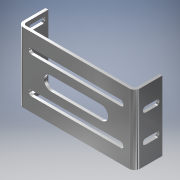
# Autodesk Inventor part: palmrest_cup
Saved by Autodesk Inventor 2018 (Build 220112000, 112)
## iProperties
Created: 2018-04-07
Part Number: palmrest_cup
Material: アルミニウム 6061
Document SubType Name: Sheet Metal
Designer: NaMACHAN
Density: 2.7 g/cm^3
Sheet Metal Rule: Default_mm
Appearance: アルミニウム - フラット
Mass: 33.0555 g
Surface Area: 100.911 cm^2
Volume: 12.2428 cm^3
Flat Pattern Width: 5 cm
Flat Pattern Length: 11.7048 cm
Flat Pattern Area: 58.5239 cm^2
Sheet Metal Width: 50.000 mm
Sheet Metal Length: 117.048 mm
Sheet Metal Area: 5852.389 mm^2
Author: NaMACHAN
Autodesk Inventor part; units mm, degrees
ref_plane "YZ Plane" through (0, 0, 0) normal (1, 0, 0) x (0, 1, 0)
ref_plane "XZ Plane" through (0, 0, 0) normal (0, 1, 0) x (-1, 0, 0)
ref_plane "XY Plane" through (0, 0, 0) normal (0, 0, 1) x (1, 0, 0)
sketch "スケッチ1" plane through (0, 0, 0) normal (0, 1, 0) x (-1, 0, 0)
  line L0 (-42, -25) -> (42, -25)
  line L1 (42, -25) -> (42, 25)
  line L2 (42, 25) -> (-42, 25)
  line L3 (-42, 25) -> (-42, -25)
  line L4 (-42, -25) -> (42, 25) construction
  line L5 (42, -25) -> (-42, 25) construction
  point P0 (0, 0)
  dimension "d0" = 84
  dimension "d1" = 50
  measures "d0" distance of L2.end L1.end
  measures "d1" distance of L1.end L0.end
extrude "プレート1" add sketch "スケッチ1" along normal blind 2
sketch "スケッチ2" plane through (-42, 0, -25) normal (-1, 0, 0) x (0, 0, 1)
  line L0 (0, 0) -> (50, 0)
  line L1 (50, 0) -> (0, 0)
  line L2 (0, 0) -> (0, 20)
  line L3 (0, 20) -> (50, 20)
  line L4 (50, 20) -> (50, 0)
  point P0 (25, 0)
  dimension "d3" = 20
  measures "d3" distance of L0.start L2.end
sheet face with bend "面2" sketch "スケッチ2" thickness 2 toward (1, 0, 0) bend radius 2
bend "曲げ1"
sketch "スケッチ3" plane through (42, 0, 25) normal (1, 0, 0) x (0, 0, -1)
  line L0 (0, 0) -> (50, 0)
  line L1 (50, 0) -> (50, 20)
  line L2 (50, 20) -> (0, 20)
  line L3 (0, 20) -> (0, 0)
  point P0 (25, 0)
  point P1 (50, 0)
  dimension "d9" = 20
  measures "d9" distance of L1.end L0.end
sheet face with bend "面3" sketch "スケッチ3" thickness 2 toward (-1, 0, 0) bend radius 2
bend "曲げ2"
sketch "スケッチ4" plane through (0, 2, 0) normal (0, 1, 0) x (1, 0, 0)
  line L0 (-32, -15) -> (32, -15)
  arc A0 (32, -15) -> (32, -11) centre (32, -13) ccw
  line L1 (32, -11) -> (-32, -11)
  arc A1 (-32, -11) -> (-32, -15) centre (-32, -13) ccw
  line L2 (-18, -5) -> (18, -5)
  arc A2 (18, -5) -> (18, 5) centre (18, 0) ccw
  line L3 (18, 5) -> (-18, 5)
  arc A3 (-18, 5) -> (-18, -5) centre (-18, 0) ccw
  line L4 (-32, 11) -> (32, 11)
  arc A4 (32, 11) -> (32, 15) centre (32, 13) ccw
  line L5 (32, 15) -> (-32, 15)
  arc A5 (-32, 15) -> (-32, 11) centre (-32, 13) ccw
  line L6 (38, -25) -> (-38, -25) projected
  line L7 (38, -25) -> (38, 25) projected
  line L8 (-38, 25) -> (-38, -25) projected
  line L9 (-38, 25) -> (38, 25) projected
  point P0 (0, 0)
  dimension "d15" = 2
  dimension "d16" = 2
  dimension "d17" = 12
  dimension "d18" = 6
  dimension "d19" = 6
  dimension "d20" = 6
  dimension "d21" = 6
  dimension "d22" = 12
  dimension "d23" = 20
  dimension "d24" = 20
  dimension "d25" = 10
  constraints: 12 end point, 12 point on circle, 12 tangent, 6 centre point, 3 horizontal, 3 parallel, 1 horizontal alignment
  measures "d15" radius of A1
  measures "d16" radius of A5
  measures "d17" distance from line of L6 A1.centre
  measures "d18" distance from line of L7 A0.centre
  measures "d19" distance from line of L8 A1.centre
  measures "d20" distance from line of L8 A5.centre
  measures "d21" distance from line of L7 A4.centre
  measures "d22" distance from line of L9 A5.centre
  measures "d23" distance from line of L8 A3.centre
  measures "d24" distance from line of L7 A2.centre
  measures "d25" distance between parallel lines of L3 L2
extrude "押し出し1" cut sketch "スケッチ4" against normal blind 10 contours A1 L1 A0 L0 | A3 L3 A2 L2 | A5 L5 A4 L4
sketch "スケッチ5" plane through (-42, 0, -25) normal (-1, 0, 0) x (0, 0, 1)
  line L0 (3, 16) -> (3, 8)
  arc A0 (3, 8) -> (7, 8) centre (5, 8) ccw
  line L1 (7, 8) -> (7, 16)
  arc A1 (7, 16) -> (3, 16) centre (5, 16) ccw
  line L2 (43, 16) -> (43, 8)
  arc A2 (43, 8) -> (47, 8) centre (45, 8) ccw
  line L3 (47, 8) -> (47, 16)
  arc A3 (47, 16) -> (43, 16) centre (45, 16) ccw
  line L4 (50, 4) -> (50, 20) projected
  line L5 (0, 20) -> (0, 4) projected
  line L6 (50, 20) -> (0, 20) projected
  line L7 (50, 4) -> (0, 4) projected
  point P0 (25, 0)
  dimension "d28" = 2
  dimension "d29" = 2
  dimension "d30" = 5
  dimension "d31" = 5
  dimension "d32" = 4
  dimension "d33" = 4
  dimension "d34" = 4
  dimension "d35" = 4
  constraints: 8 end point, 8 point on circle, 8 tangent, 4 centre point, 2 parallel, 2 vertical
  measures "d28" radius of A1
  measures "d29" radius of A3
  measures "d30" distance from line of L4 A3.centre
  measures "d31" distance from line of L5 A1.centre
  measures "d32" distance from line of L6 A1.centre
  measures "d33" distance from line of L7 A0.centre
  measures "d34" distance from line of L7 A2.centre
  measures "d35" distance from line of L6 A3.centre
extrude "押し出し2" cut sketch "スケッチ5" against normal blind 10 contours A1 L1 A0 L0 | A3 L3 A2 L2
sketch "スケッチ6" plane through (42, 0, 25) normal (1, 0, 0) x (0, 0, -1)
  line L0 (13, 16) -> (13, 8)
  arc A0 (13, 8) -> (17, 8) centre (15, 8) ccw
  line L1 (17, 8) -> (17, 16)
  arc A1 (17, 16) -> (13, 16) centre (15, 16) ccw
  line L2 (33, 16) -> (33, 8)
  arc A2 (33, 8) -> (37, 8) centre (35, 8) ccw
  line L3 (37, 8) -> (37, 16)
  arc A3 (37, 16) -> (33, 16) centre (35, 16) ccw
  line L4 (50, 4) -> (50, 20) projected
  line L5 (0, 20) -> (0, 4) projected
  line L6 (50, 20) -> (0, 20) projected
  line L7 (50, 4) -> (0, 4) projected
  point P0 (25, 0)
  dimension "d38" = 2
  dimension "d39" = 2
  dimension "d40" = 15
  dimension "d41" = 15
  dimension "d42" = 4
  dimension "d43" = 4
  constraints: 8 end point, 8 point on circle, 6 tangent, 4 centre point, 4 horizontal alignment, 2 parallel, 2 vertical
  measures "d38" radius of A1
  measures "d39" radius of A3
  measures "d40" distance from line of L4 A3.centre
  measures "d41" distance from line of L5 A1.centre
  measures "d42" distance from line of L6 A1.centre
  measures "d43" distance from line of L7 A0.centre
extrude "押し出し3" cut sketch "スケッチ6" against normal blind 10 contours A1 L1 A0 L0 | A3 L3 A2 L2
equation "\"d2\" = Thickness"
equation "\"d4\" = BendRadius"
equation "\"d5\" = BendReliefWidth"
equation "\"d7\" = MinimumRemnant"
equation "\"d6\" = BendReliefDepth"
equation "\"d8\" = TransitionRadius"
equation "\"d10\" = BendRadius"
equation "\"d11\" = BendReliefWidth"
equation "\"d13\" = MinimumRemnant"
equation "\"d12\" = BendReliefDepth"
equation "\"d14\" = TransitionRadius"
equation "\"BendRadius\" = Thickness"
equation "\"BendReliefWidth\" = Thickness"
equation "\"BendReliefDepth\" = 0.5 * Thickness"
equation "\"CornerReliefSize\" = 4 * Thickness"
equation "\"MinimumRemnant\" = 2 * Thickness"
equation "\"TransitionRadius\" = BendRadius"
equation "\"JacobiRadiusSize\" = BendRadius"
equation "\"GapSize\" = Thickness"
equation "\"Thickness\" = 2"
